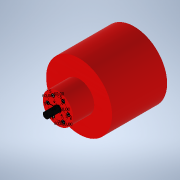
# Autodesk Inventor part: Motor
Saved by Autodesk Inventor 2020.3 (Build 243373010, 373A)
## iProperties
Created: 2020-02-14
Part Number: Motor
Material: Generisch
Document SubType Name: Modeling
Designer: Stefan
Density: 1 g/cm^3
Appearance: Vorgabe
Mass: 922.695 g
Surface Area: 598.992 cm^2
Volume: 922.695 cm^3
Author: Stefan
Autodesk Inventor part; units mm, degrees
ref_plane "YZ Plane" through (0, 0, 0) normal (1, 0, 0) x (0, 1, 0)
ref_plane "XZ Plane" through (0, 0, 0) normal (0, 1, 0) x (-1, 0, 0)
ref_plane "XY Plane" through (0, 0, 0) normal (0, 0, 1) x (1, 0, 0)
sketch "Skizze1" plane through (0, 0, 0) normal (0, 0, 1) x (1, 0, 0)
  circle A0 centre (0, 0) radius 54.5
  dimension "d0" = 109
  constraints: 1 centre point, 1 coincident
  measures "d0" diameter of A0
extrude "Extrusion1" add sketch "Skizze1" along normal blind 91
sketch "Skizze2" plane through (0, 0, 0) normal (0, 0, -1) x (-1, 0, 0)
  circle A0 centre (35, -35) radius 2.5
  circle A1 centre (-35, -35) radius 2.5
  circle A2 centre (-35, 35) radius 2.5
  circle A3 centre (35, 35) radius 2.5
  point P0 (0, 0)
  dimension "d15" = 5
  dimension "d16" = 5
  dimension "d17" = 5
  dimension "d18" = 5
  dimension "d19" = 35
  dimension "d20" = 35
  dimension "d21" = 35
  dimension "d22" = 35
  dimension "d23" = 35
  dimension "d24" = 35
  dimension "d25" = 35
  dimension "d26" = 35
  constraints: 4 centre point
  measures "d15" diameter of A0
  measures "d16" diameter of A1
  measures "d17" diameter of A2
  measures "d18" diameter of A3
  measures "d19" horizontal distance of point (0, 0) A0.centre
  measures "d20" horizontal distance of point (0, 0) A0.centre
  measures "d21" horizontal distance of point (0, 0) A1.centre
  measures "d22" horizontal distance of point (0, 0) A1.centre
  measures "d23" horizontal distance of point (0, 0) A2.centre
  measures "d24" horizontal distance of A2.centre point (0, 0)
  measures "d25" horizontal distance of A3.centre point (0, 0)
  measures "d26" horizontal distance of point (0, 0) A3.centre
sketch "Skizze3" plane through (0, 0, 91) normal (0, 0, 1) x (1, 0, 0)
  circle A0 centre (0, 0) radius 25
  dimension "d29" = 50
  constraints: 1 centre point, 1 coincident
  measures "d29" diameter of A0
extrude "Extrusion3" add sketch "Skizze3" along normal blind 35
sketch "Skizze4" plane through (0, 0, 126) normal (0, 0, 1) x (1, 0, 0)
  circle A0 centre (0, 0) radius 4.95
  circle A1 centre (0, 0) radius 17 construction
  line L0 (0, 0) -> (-17, 0)
  line L1 (0, 0) -> (-8.5, 14.7224) construction
  line L2 (0, 0) -> (8.5, 14.7224) construction
  line L3 (0, 0) -> (17, 0) construction
  line L4 (0, 0) -> (8.5, -14.7224) construction
  circle A2 centre (8.5, -14.7224) radius 2.5
  circle A3 centre (-17, 0) radius 2.5
  circle A4 centre (-8.5, 14.7224) radius 2.5
  circle A5 centre (8.5, 14.7224) radius 2.5
  circle A6 centre (17, 0) radius 2.5
  line L5 (-8.5, -14.7224) -> (0, 0) construction
  circle A7 centre (-8.5, -14.7224) radius 2.5
  dimension "d32" = 9.9
  dimension "d33" = 34
  dimension "d34" = 60
  dimension "d35" = 60
  dimension "d36" = 60
  dimension "d37" = 60
  dimension "d38" = 5
  dimension "d39" = 5
  dimension "d40" = 5
  dimension "d41" = 5
  dimension "d42" = 5
  dimension "d45" = 5
  dimension "d46" = 60
  constraints: 12 end point, 8 centre point, 8 coincident, 6 point on circle, 1 horizontal
  measures "d32" diameter of A0
  measures "d33" diameter of A1
  measures "d34" angle of L1 L0
  measures "d35" angle of L2 L1
  measures "d36" angle of L3 L2
  measures "d37" angle of L4 L3
  measures "d38" diameter of A2
  measures "d39" diameter of A3
  measures "d40" diameter of A4
  measures "d41" diameter of A5
  measures "d42" diameter of A6
  measures "d45" diameter of A7
  measures "d46" angle of L4 L5
hole "Bohrung1" at (35, 35, 0) direction (0, 0, 1) diameter 4.917 depth 13 tip angle 118 thread size "M6x1" class "6H" standard "ISO Metric profile"
hole "Bohrung2" at (35, -35, 0) direction (0, 0, 1) diameter 4.917 depth 13 tip angle 118 thread size "M6x1" class "6H" standard "ISO Metric profile"
hole "Bohrung3" at (-35, -35, 0) direction (0, 0, 1) diameter 4.917 depth 13 tip angle 118 thread size "M6x1" class "6H" standard "ISO Metric profile"
hole "Bohrung4" at (-35, 35, 0) direction (0, 0, 1) diameter 4.917 depth 13 tip angle 118 thread size "M6x1" class "6H" standard "ISO Metric profile"
extrude "Extrusion5" add sketch "Skizze4" along normal blind 20 contours A0
hole "Bohrung17" at (8.5, 14.7224, 126) direction (0, 0, -1) diameter 4.134 depth 8 tip angle 118 thread size "M5x0.8" class "6H" standard "ISO Metric profile"
pattern_circular "Runde Anordnung1" count 6 over 360 about axis through (0, 0, 126) along (0, 0, 1) of "Bohrung17"
